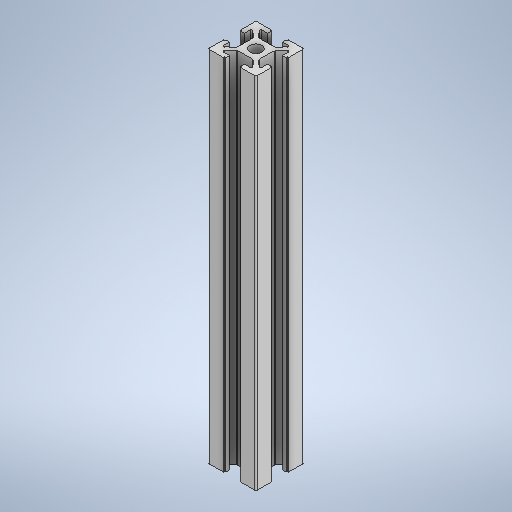
# Autodesk Inventor part: Peça3
Saved by Autodesk Inventor 2025.2 (Build 292293000, 293)
## iProperties
Created: 2025-04-04
Part Number: Peça3
Material: Genérico
Document SubType Name: Sheet Metal
Designer: kenay
Density: 1 g/cm^3
Sheet Metal Rule: Padrão_mm
Appearance: Padrão
Author: kenay
Autodesk Inventor part; units mm, degrees
ref_plane "YZ Plane" through (0, 0, 0) normal (1, 0, 0) x (0, 1, 0)
ref_plane "XZ Plane" through (0, 0, 0) normal (0, 1, 0) x (-1, 0, 0)
ref_plane "XY Plane" through (0, 0, 0) normal (0, 0, 1) x (1, 0, 0)
sketch "Esboço1" plane through (0, 0, 0) normal (0, 1, 0) x (-1, 0, 0)
  line L0 (-10, 10) -> (10, 10) construction
  line L1 (10, 10) -> (10, -10) construction
  line L2 (10, -10) -> (-10, -10) construction
  line L3 (-10, -10) -> (-10, 10) construction
  line L4 (-10, 10) -> (10, -10) construction
  line L5 (10, 10) -> (-10, -10) construction
  line L6 (0, -4.5) -> (3.1, -4.5)
  line L7 (0, -10) -> (0, 10) construction
  line L8 (5.8739, -7.1527) -> (3.4597, -4.6527)
  arc A0 (3.4597, -4.6527) -> (3.1, -4.5) centre (3.1, -5) ccw
  line L9 (5.5142, -8) -> (3.1, -8)
  arc A1 (5.5142, -8) -> (5.8739, -7.1527) centre (5.5142, -7.5) ccw
  line L10 (3.1, -9.5) -> (3.1, -8)
  line L11 (3.6, -9.5) -> (3.1, -9.5)
  line L12 (3.6, -10) -> (3.6, -9.5)
  line L13 (10, -10) -> (3.6, -10) construction
  line L14 (10, -10) -> (0, -10) construction
  line L15 (10, -10) -> (10, -3.6) construction
  line L16 (9.5, -3.1) -> (8, -3.1)
  line L17 (9.5, -3.1) -> (9.5, -3.6)
  line L18 (9.5, -3.6) -> (10, -3.6)
  line L19 (8, -3.1) -> (8, -5.5142)
  line L20 (7.1527, -5.8739) -> (4.6527, -3.4597)
  line L21 (4.5, 0) -> (4.5, -3.1)
  arc A2 (4.5, -3.1) -> (4.6527, -3.4597) centre (5, -3.1) ccw
  line L22 (10, 0) -> (0, 0) construction
  line L23 (4.5, 0) -> (2.5, 0)
  line L24 (0, -4.5) -> (0, -2.5)
  arc A3 (7.1527, -5.8739) -> (8, -5.5142) centre (7.5, -5.5142) ccw
  arc A4 (0, -2.5) -> (2.5, 0) centre (0, 0) ccw
  arc A5 (9.5, -10) -> (10, -9.5) centre (9.5, -9.5) ccw
  line L25 (9.5, -10) -> (3.6, -10)
  line L26 (10, -9.5) -> (10, -3.6)
  point P0 (3.5, 0)
  dimension "d0" = 20
  dimension "d5" = 0.5
  dimension "d6" = 1
  dimension "d7" = 0.5
  dimension "d8" = 2
  dimension "d10" = 6.9
  dimension "d12" = 3.1
  dimension "d15" = 2.5
  dimension "d16" = 2
  constraints: 54 end point, 12 point on circle, 10 equal length, 9 tangent, 8 horizontal, 7 point on line, 6 centre point, 6 midpoint, 6 vertical, 3 collinear, 3 equal radius, 2 parallel, 2 perpendicular, 1 coincident, 1 other
  measures "d0" distance between parallel lines of L3 L1
  measures "d5" radius of A0
  measures "d6" angle of L4 L8
  measures "d7" distance of L10.start L11.start
  measures "d8" distance between parallel lines of L13 L9
  measures "d10" distance between parallel lines of L1 L10
  measures "d12" distance of L21.start L21.end
  measures "d15" radius of A4
  measures "d16" distance of L23.end L21.start
extrude "Extrusão1" add sketch "Esboço1" along normal mid plane 150
mirror "Espelhar1" about plane through (0, 0, 0) normal (1, 0, 0) of "Extrusão1"
mirror "Espelhar2" about plane through (0, 0, 0) normal (0, 0, 1) of "Extrusão1", "Espelhar1"
equation "\"Raio_vergadura\" = Espessura"
equation "\"Largura_alívio_de_vergadura\" = Espessura"
equation "\"Profundidade_alívio_de_vergadura\" = 0.5 * Espessura"
equation "\"Tamanho_alívio_de_dobra\" = 4 * Espessura"
equation "\"Remanescente_mínimo\" = 2 * Espessura"
equation "\"Raiodetransição\" = Raio_vergadura"
equation "\"Tamanho_de_raio_de_Jacobi\" = Raio_vergadura"
equation "\"TamanhoFolga\" = Espessura"
equation "\"Espessura\" = 0.5"
